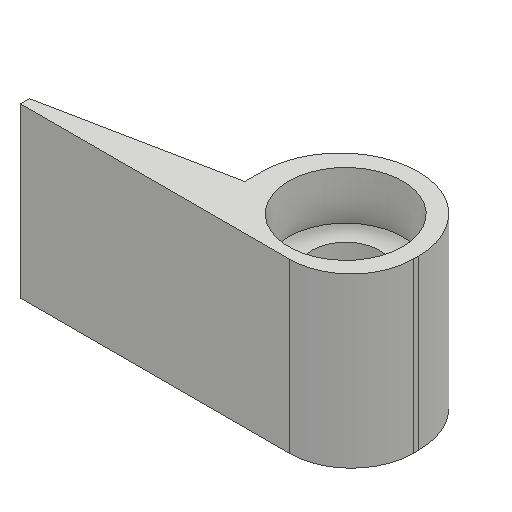
# Autodesk Inventor part: 3DP_PLA_Front_blade_hinge
Saved by Autodesk Inventor 2025 (Build 290162010, 162A)
## iProperties
Created: 2016-05-09
Part Number: 3DP_PLA_Front_blade_hinge
Material: Ogólny
Document SubType Name: Modeling
Designer: Andrzej
Density: 1 g/cm^3
Appearance: Domyślna
Mass: 1.7551 g
Surface Area: 18.1576 cm^2
Volume: 1.7551 cm^3
Author: Andrzej
Autodesk Inventor part; units mm, degrees
ref_plane "YZ Plane" through (0, 0, 0) normal (1, 0, 0) x (0, 1, 0)
ref_plane "XZ Plane" through (0, 0, 0) normal (0, 1, 0) x (-1, 0, 0)
ref_plane "XY Plane" through (0, 0, 0) normal (0, 0, 1) x (1, 0, 0)
sketch "Szkic1" plane through (0, 0, 0) normal (0, 0, 1) x (1, 0, 0)
  line L0 (-2.9617, 9.0824) -> (-2.9617, 9.0824)
  line L1 (-9.9617, 2.0824) -> (-9.9617, -3.4176)
  line L2 (-9.9617, -3.4176) -> (-1.9617, -3.4176)
  line L3 (3.5383, 2.0824) -> (3.5383, 2.5824)
  circle A0 centre (-2.9617, 2.5824) radius 5.075
  arc A1 (-2.9617, 9.0824) -> (-9.9617, 2.0824) centre (-2.9617, 2.0824) ccw
  arc A2 (3.5383, 2.5824) -> (-2.9617, 9.0824) centre (-2.9617, 2.5824) ccw
  arc A3 (-1.9617, -3.4176) -> (3.5383, 2.0824) centre (-1.9617, 2.0824) ccw
  line L4 (-9.9617, -3.4176) -> (-25.9617, -3.4176)
  line L5 (-25.9617, -3.4176) -> (-25.9617, -2.6176)
  line L6 (-25.9617, -2.6176) -> (-9.9617, 0.5824)
  point P0 (0, 0)
  point P1 (3.5383, 9.0824)
  point P2 (-9.9617, 9.0824)
  point P3 (3.5383, -3.4176)
  dimension "d3" = 13.5
  dimension "d4" = 12.5
  dimension "d7" = 6.5
  dimension "d8" = 7
  dimension "d9" = 10.15
  dimension "d10" = 7
  dimension "d11" = 6.5
  dimension "d12" = 5.5
  dimension "d13" = 16
  dimension "d46" = 0.8
  dimension "d47" = 1.5
  constraints: 14 end point, 7 point on circle, 7 point on line, 6 tangent, 4 centre point, 2 parallel, 1 coincident, 1 horizontal, 1 perpendicular, 1 vertical
  measures "d3" distance of point (3.538, 9.082) point (-9.962, 9.082)
  measures "d4" distance of point (-9.962, 9.082) L1.end
  measures "d7" distance from line of L0 point (-2.962, 2.582)
  measures "d8" distance from line of L1 point (-2.962, 2.582)
  measures "d9" diameter of A0
  measures "d10" radius of A1
  measures "d11" radius of A2
  measures "d12" radius of A3
  measures "d13" distance of L1.end L4.end
  measures "d46" distance of L4.end L5.end
  measures "d47" distance of L1.start L6.end
extrude "Wyciągnięcie proste1" add sketch "Szkic1" along normal blind 15 contours A1 A2 L3 A3 L2 L1 | L1 L4 L5 L6 | A0
extrude "Wyciągnięcie proste2" cut sketch "Szkic1" along normal blind 5.9 contours A0
hole "Otwór1" at (-2.9617, 2.5824, 0) direction (0, 0, 1) diameter 6 end through all
sketch "Szkic2" plane through (0, 0, 15) normal (0, 0, 1) x (1, 0, 0)
  circle A0 centre (-2.9617, 2.5824) radius 5.075 projected
  point P0 (0, 0)
extrude "Wyciągnięcie proste3" cut sketch "Szkic2" against normal blind 4.3
ref_plane "Płaszczyzna konstrukcyjna1" through (-25.9617, 11.5824, 0) normal (0, -1, 0) x (1, 0, 0)
